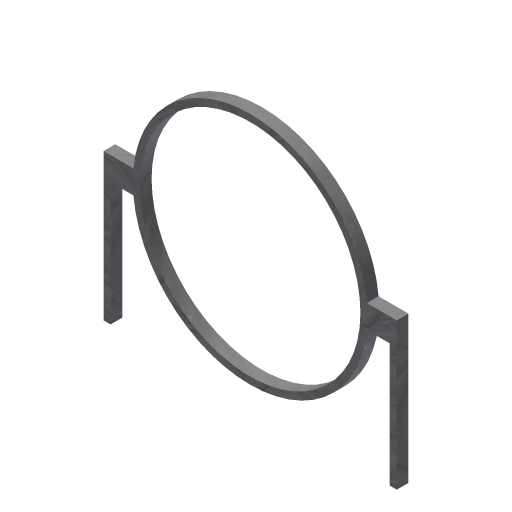
# Autodesk Inventor part: PIEZA_JACLUBER_2
Saved by Autodesk Inventor 2024.3 (Build 283343000, 343)
## iProperties
Created: 2024-06-21
Part Number: PIEZA_JACLUBER_2
Material: Steel, Mild, Welded
Document SubType Name: Modeling
Designer: Niler
Density: 7.85 g/cm^3
Appearance: Weld - Steel Mild
Author: Niler
Autodesk Inventor part; units mm, degrees
ref_plane "YZ Plane" through (0, 0, 0) normal (1, 0, 0) x (0, 1, 0)
ref_plane "XZ Plane" through (0, 0, 0) normal (0, 1, 0) x (-1, 0, 0)
ref_plane "XY Plane" through (0, 0, 0) normal (0, 0, 1) x (1, 0, 0)
sketch "Sketch1" plane through (0, 0, 0) normal (0, 0, 1) x (1, 0, 0)
  circle A0 centre (0, 0) radius 50
  circle A1 centre (0, 0) radius 47
  line L0 (37.5, 5) -> (62.5, 5)
  line L1 (62.5, 5) -> (62.5, -5)
  line L2 (62.5, -5) -> (37.5, -5)
  line L3 (37.5, -5) -> (37.5, 5)
  line L4 (37.5, 5) -> (62.5, -5) construction
  line L5 (62.5, 5) -> (37.5, -5) construction
  line L6 (-62.5, 5) -> (-37.5, 5)
  line L7 (-37.5, 5) -> (-37.5, -5)
  line L8 (-37.5, -5) -> (-62.5, -5)
  line L9 (-62.5, -5) -> (-62.5, 5)
  line L10 (-62.5, 5) -> (-37.5, -5) construction
  line L11 (-37.5, 5) -> (-62.5, -5) construction
  line L12 (62.5, 0) -> (59.5, 0)
  line L13 (59.5, 0) -> (59.5, -57.5)
  line L14 (59.5, -57.5) -> (62.5, -57.5)
  line L15 (62.5, -57.5) -> (62.5, 0)
  line L16 (-62.5, 0) -> (-59.5, 0)
  line L17 (-59.5, 0) -> (-59.5, -57.5)
  line L18 (-59.5, -57.5) -> (-62.5, -57.5)
  line L19 (-62.5, -57.5) -> (-62.5, 0)
  point P0 (50, 0)
  point P1 (-50, 0)
  point P2 (49.7494, 5)
  point P3 (-49.7494, 5)
  point P4 (-59.5, -5)
  point P5 (-49.7494, -5)
  point P6 (49.7494, -5)
  point P7 (59.5, -5)
  dimension "d0" = 100
  dimension "d1" = 94
  dimension "d2" = 25
  dimension "d3" = 10
  dimension "d4" = 25
  dimension "d5" = 10
  dimension "d6" = 3
  dimension "d7" = 57.5
  dimension "d8" = 3
  dimension "d9" = 57.5
  constraints: 40 end point, 8 parallel, 6 midpoint, 4 horizontal, 4 perpendicular, 2 centre point, 2 coincident, 2 point on circle
  measures "d0" diameter of A0
  measures "d1" diameter of A1
  measures "d2" distance of L1.end L2.end
  measures "d3" distance of L0.end L1.end
  measures "d4" distance of L7.end L8.end
  measures "d5" distance of L6.end L7.end
  measures "d6" distance of L14.end L13.end
  measures "d7" distance of L13.end L12.end
  measures "d8" distance of L17.end L18.end
  measures "d9" distance of L16.end L17.end
extrude "Extrusion1" add sketch "Sketch1" along normal blind 5 contours A0 L2 A1 L0 | A0 L0 L1 L12 L13 L2 | L0 A1 L6 A0 | A0 L8 A1 L2 | L6 A1 L8 A0 | A0 L8 L17 L16 L9 L6 | L13 L12 L1 L2 | L2 L15 L14 L13 | L17 L18 L19 L8 | L8 L9 L16 L17
body "Solid1"
